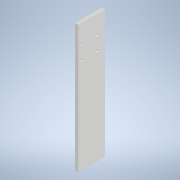
# Autodesk Inventor part: 縦フラットバー
Saved by Autodesk Inventor 2022 (Build 260153000, 153)
## iProperties
Created: 2022-10-17
Part Number: 縦フラットバー
Material: アルミニウム
Document SubType Name: Modeling
Designer: tdn82
Density: 2.7 g/cm^3
Appearance: サテン
Author: tdn82
Autodesk Inventor part; units mm, degrees
ref_plane "YZ Plane" through (0, 0, 0) normal (1, 0, 0) x (0, 1, 0)
ref_plane "XZ Plane" through (0, 0, 0) normal (0, 1, 0) x (-1, 0, 0)
ref_plane "XY Plane" through (0, 0, 0) normal (0, 0, 1) x (1, 0, 0)
sketch "スケッチ1" plane through (0, 0, 0) normal (0, 1, 0) x (-1, 0, 0)
  line L0 (0, 0) -> (-5, 0)
  line L1 (-5, 0) -> (-5, -40)
  line L2 (-5, -40) -> (0, -40)
  line L3 (0, -40) -> (0, 0)
  dimension "d0" = 40
  dimension "d3" = 5
  constraints: 8 end point, 2 parallel, 1 horizontal, 1 perpendicular
  measures "d0" distance of L2.end L0.start
  measures "d3" distance of L0.start L0.end
extrude "押し出し1" add sketch "スケッチ1" along normal blind 190
sketch "スケッチ2" plane through (5, 0, 0) normal (1, 0, 0) x (0, 0, -1)
  line L0 (0, 0) -> (0, 190) projected
  line L1 (0, 190) -> (40, 190) projected
  line L2 (0, 0) -> (0, 190) projected
  line L3 (40, 0) -> (40, 190) projected
  line L4 (0, 95) -> (40, 95)
  point P0 (4, 163)
  point P1 (28, 163)
  point P2 (4, 143)
  point P3 (28, 143)
  dimension "d4" = 4
  dimension "d5" = 27
  dimension "d8" = 24
  dimension "d11" = 20
  constraints: 2 end point, 2 midpoint, 1 horizontal, 1 vertical, 3 other
  measures "d4" distance from line of point (4, 163) L0
  measures "d5" distance from line of point (4, 163) L1
  measures "d8" distance of point (4, 163) point (28, 163)
  measures "d11" distance of point (4, 163) point (4, 143)
hole "穴1" at (5, 163, -4) at (5, 163, -28) at (5, 143, -4) at (5, 143, -28) direction (-1, 0, 0) diameter 3.5 end through all
